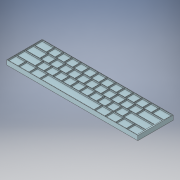
# Autodesk Inventor part: keyboard-base_standard
Saved by Autodesk Inventor 2016 (Build 200138000, 138)
## iProperties
Created: 2016-12-08
Part Number: keyboard-base_standard
Material: Generic
Document SubType Name: Modeling
Designer: Cemra JC
Density: 1 g/cm^3
Appearance: Default
Author: Cemra JC
Autodesk Inventor part; units mm, degrees
ref_plane "YZ Plane" through (0, 0, 0) normal (1, 0, 0) x (0, 1, 0)
ref_plane "XZ Plane" through (0, 0, 0) normal (0, 1, 0) x (-1, 0, 0)
ref_plane "XY Plane" through (0, 0, 0) normal (0, 0, 1) x (1, 0, 0)
sketch "Keyboard Backplane" plane through (0, 0, 0) normal (0, 1, 0) x (-1, 0, 0)
  line L0 (144, 38.9) -> (-144, 38.9)
  line L1 (-144, 38.9) -> (-144, -38.9)
  line L2 (-144, -38.9) -> (144, -38.9)
  line L3 (144, -38.9) -> (144, 38.9)
  line L4 (144, 38.9) -> (-144, -38.9) construction
  line L5 (-144, 38.9) -> (144, -38.9) construction
  point P0 (0, 0)
  point P1 (0, 0)
  dimension "d0" = 77.8
  dimension "d1" = 288
  constraints: 12 end point, 2 parallel, 1 coincident, 1 horizontal, 1 midpoint, 1 perpendicular
  measures "d0" distance of L0.end L1.end
  measures "d1" distance of L1.end L2.end
extrude "Keyboard Backplane Body" add sketch "Keyboard Backplane" along normal blind 10
sketch "KeyCap Outlines" plane through (0, 10, 0) normal (0, 1, 0) x (1, 0, 0)
  line L0 (-143, 37.9) -> (-115.7, 37.9)
  line L1 (-115.7, 37.9) -> (-115.7, 19.7)
  line L2 (-115.7, 19.7) -> (-143, 19.7)
  line L3 (-143, 19.7) -> (-143, 37.9)
  line L4 (-144, -38.9) -> (144, -38.9) projected
  line L5 (144, -38.9) -> (144, 38.9) projected
  line L6 (144, 38.9) -> (-144, 38.9) projected
  line L7 (-144, 38.9) -> (-144, -38.9) projected
  line L8 (-114.7, 19.7) -> (-96.5, 19.7)
  line L9 (-96.5, 19.7) -> (-96.5, 37.9)
  line L10 (-96.5, 37.9) -> (-114.7, 37.9)
  line L11 (-114.7, 37.9) -> (-114.7, 19.7)
  line L12 (-95.5, 19.7) -> (-77.3, 19.7)
  line L13 (-77.3, 19.7) -> (-77.3, 37.9)
  line L14 (-77.3, 37.9) -> (-95.5, 37.9)
  line L15 (-95.5, 37.9) -> (-95.5, 19.7)
  line L16 (-76.3, 19.7) -> (-58.1, 19.7)
  line L17 (-58.1, 19.7) -> (-58.1, 37.9)
  line L18 (-58.1, 37.9) -> (-76.3, 37.9)
  line L19 (-76.3, 37.9) -> (-76.3, 19.7)
  line L20 (-57.1, 19.7) -> (-38.9, 19.7)
  line L21 (-38.9, 19.7) -> (-38.9, 37.9)
  line L22 (-38.9, 37.9) -> (-57.1, 37.9)
  line L23 (-57.1, 37.9) -> (-57.1, 19.7)
  line L24 (-37.9, 19.7) -> (-19.7, 19.7)
  line L25 (-19.7, 19.7) -> (-19.7, 37.9)
  line L26 (-19.7, 37.9) -> (-37.9, 37.9)
  line L27 (-37.9, 37.9) -> (-37.9, 19.7)
  line L28 (-18.7, 19.7) -> (-0.5, 19.7)
  line L29 (-0.5, 19.7) -> (-0.5, 37.9)
  line L30 (-0.5, 37.9) -> (-18.7, 37.9)
  line L31 (-18.7, 37.9) -> (-18.7, 19.7)
  line L32 (0.5, 19.7) -> (18.7, 19.7)
  line L33 (18.7, 19.7) -> (18.7, 37.9)
  line L34 (18.7, 37.9) -> (0.5, 37.9)
  line L35 (0.5, 37.9) -> (0.5, 19.7)
  line L36 (19.7, 19.7) -> (37.9, 19.7)
  line L37 (37.9, 19.7) -> (37.9, 37.9)
  line L38 (37.9, 37.9) -> (19.7, 37.9)
  line L39 (19.7, 37.9) -> (19.7, 19.7)
  line L40 (38.9, 19.7) -> (57.1, 19.7)
  line L41 (57.1, 19.7) -> (57.1, 37.9)
  line L42 (57.1, 37.9) -> (38.9, 37.9)
  line L43 (38.9, 37.9) -> (38.9, 19.7)
  line L44 (58.1, 19.7) -> (76.3, 19.7)
  line L45 (76.3, 19.7) -> (76.3, 37.9)
  line L46 (76.3, 37.9) -> (58.1, 37.9)
  line L47 (58.1, 37.9) -> (58.1, 19.7)
  line L48 (77.3, 19.7) -> (95.5, 19.7)
  line L49 (95.5, 19.7) -> (95.5, 37.9)
  line L50 (95.5, 37.9) -> (77.3, 37.9)
  line L51 (77.3, 37.9) -> (77.3, 19.7)
  line L52 (96.5, 19.7) -> (114.7, 19.7)
  line L53 (114.7, 19.7) -> (114.7, 37.9)
  line L54 (114.7, 37.9) -> (96.5, 37.9)
  line L55 (96.5, 37.9) -> (96.5, 19.7)
  line L56 (115.7, 37.9) -> (143, 37.9)
  line L57 (143, 37.9) -> (143, 19.7)
  line L58 (143, 19.7) -> (115.7, 19.7)
  line L59 (115.7, 19.7) -> (115.7, 37.9)
  line L60 (-143, 18.7) -> (-111.15, 18.7)
  line L61 (-111.15, 18.7) -> (-111.15, 0.5)
  line L62 (-111.15, 0.5) -> (-143, 0.5)
  line L63 (-143, 0.5) -> (-143, 18.7)
  line L64 (-110.15, 0.5) -> (-91.95, 0.5)
  line L65 (-91.95, 0.5) -> (-91.95, 18.7)
  line L66 (-91.95, 18.7) -> (-110.15, 18.7)
  line L67 (-110.15, 18.7) -> (-110.15, 0.5)
  line L68 (-72.75, 0.5) -> (-72.75, 18.7)
  line L69 (-72.75, 18.7) -> (-90.95, 18.7)
  line L70 (-90.95, 18.7) -> (-90.95, 0.5)
  line L71 (-90.95, 0.5) -> (-72.75, 0.5)
  line L72 (-53.55, 0.5) -> (-53.55, 18.7)
  line L73 (-53.55, 18.7) -> (-71.75, 18.7)
  line L74 (-71.75, 18.7) -> (-71.75, 0.5)
  line L75 (-71.75, 0.5) -> (-53.55, 0.5)
  line L76 (-34.35, 0.5) -> (-34.35, 18.7)
  line L77 (-34.35, 18.7) -> (-52.55, 18.7)
  line L78 (-52.55, 18.7) -> (-52.55, 0.5)
  line L79 (-52.55, 0.5) -> (-34.35, 0.5)
  line L80 (-15.15, 0.5) -> (-15.15, 18.7)
  line L81 (-15.15, 18.7) -> (-33.35, 18.7)
  line L82 (-33.35, 18.7) -> (-33.35, 0.5)
  line L83 (-33.35, 0.5) -> (-15.15, 0.5)
  line L84 (4.05, 0.5) -> (4.05, 18.7)
  line L85 (4.05, 18.7) -> (-14.15, 18.7)
  line L86 (-14.15, 18.7) -> (-14.15, 0.5)
  line L87 (-14.15, 0.5) -> (4.05, 0.5)
  line L88 (23.25, 0.5) -> (23.25, 18.7)
  line L89 (23.25, 18.7) -> (5.05, 18.7)
  line L90 (5.05, 18.7) -> (5.05, 0.5)
  line L91 (5.05, 0.5) -> (23.25, 0.5)
  line L92 (42.45, 0.5) -> (42.45, 18.7)
  line L93 (42.45, 18.7) -> (24.25, 18.7)
  line L94 (24.25, 18.7) -> (24.25, 0.5)
  line L95 (24.25, 0.5) -> (42.45, 0.5)
  line L96 (61.65, 0.5) -> (61.65, 18.7)
  line L97 (61.65, 18.7) -> (43.45, 18.7)
  line L98 (43.45, 18.7) -> (43.45, 0.5)
  line L99 (43.45, 0.5) -> (61.65, 0.5)
  line L100 (80.85, 0.5) -> (80.85, 18.7)
  line L101 (80.85, 18.7) -> (62.65, 18.7)
  line L102 (62.65, 18.7) -> (62.65, 0.5)
  line L103 (62.65, 0.5) -> (80.85, 0.5)
  line L104 (100.05, 0.5) -> (100.05, 18.7)
  line L105 (100.05, 18.7) -> (81.85, 18.7)
  line L106 (81.85, 18.7) -> (81.85, 0.5)
  line L107 (81.85, 0.5) -> (100.05, 0.5)
  line L108 (101.05, 18.7) -> (142, 18.7)
  line L109 (142, 18.7) -> (142, 0.5)
  line L110 (142, 0.5) -> (101.05, 0.5)
  line L111 (101.05, 0.5) -> (101.05, 18.7)
  line L112 (-143, -0.5) -> (-102.05, -0.5)
  line L113 (-102.05, -0.5) -> (-102.05, -18.7)
  line L114 (-102.05, -18.7) -> (-143, -18.7)
  line L115 (-143, -18.7) -> (-143, -0.5)
  line L116 (-101.05, -0.5) -> (-82.85, -0.5)
  line L117 (-82.85, -0.5) -> (-82.85, -18.7)
  line L118 (-82.85, -18.7) -> (-101.05, -18.7)
  line L119 (-101.05, -18.7) -> (-101.05, -0.5)
  line L120 (-63.65, -18.7) -> (-81.85, -18.7)
  line L121 (-63.65, -0.5) -> (-63.65, -18.7)
  line L122 (-81.85, -18.7) -> (-81.85, -0.5)
  line L123 (-81.85, -0.5) -> (-63.65, -0.5)
  line L124 (-44.45, -18.7) -> (-62.65, -18.7)
  line L125 (-44.45, -0.5) -> (-44.45, -18.7)
  line L126 (-62.65, -18.7) -> (-62.65, -0.5)
  line L127 (-62.65, -0.5) -> (-44.45, -0.5)
  line L128 (-25.25, -18.7) -> (-43.45, -18.7)
  line L129 (-25.25, -0.5) -> (-25.25, -18.7)
  line L130 (-43.45, -18.7) -> (-43.45, -0.5)
  line L131 (-43.45, -0.5) -> (-25.25, -0.5)
  line L132 (-6.05, -18.7) -> (-24.25, -18.7)
  line L133 (-6.05, -0.5) -> (-6.05, -18.7)
  line L134 (-24.25, -18.7) -> (-24.25, -0.5)
  line L135 (-24.25, -0.5) -> (-6.05, -0.5)
  line L136 (13.15, -18.7) -> (-5.05, -18.7)
  line L137 (13.15, -0.5) -> (13.15, -18.7)
  line L138 (-5.05, -18.7) -> (-5.05, -0.5)
  line L139 (-5.05, -0.5) -> (13.15, -0.5)
  line L140 (32.35, -18.7) -> (14.15, -18.7)
  line L141 (32.35, -0.5) -> (32.35, -18.7)
  line L142 (14.15, -18.7) -> (14.15, -0.5)
  line L143 (14.15, -0.5) -> (32.35, -0.5)
  line L144 (51.55, -18.7) -> (33.35, -18.7)
  line L145 (51.55, -0.5) -> (51.55, -18.7)
  line L146 (33.35, -18.7) -> (33.35, -0.5)
  line L147 (33.35, -0.5) -> (51.55, -0.5)
  line L148 (70.75, -18.7) -> (52.55, -18.7)
  line L149 (70.75, -0.5) -> (70.75, -18.7)
  line L150 (52.55, -18.7) -> (52.55, -0.5)
  line L151 (52.55, -0.5) -> (70.75, -0.5)
  line L152 (89.95, -18.7) -> (71.75, -18.7)
  line L153 (89.95, -0.5) -> (89.95, -18.7)
  line L154 (71.75, -18.7) -> (71.75, -0.5)
  line L155 (71.75, -0.5) -> (89.95, -0.5)
  line L156 (90.95, -18.7) -> (141, -18.7)
  line L157 (141, -18.7) -> (141, -0.5)
  line L158 (141, -0.5) -> (90.95, -0.5)
  line L159 (90.95, -0.5) -> (90.95, -18.7)
  line L160 (-143, -37.9) -> (-120.25, -37.9)
  line L161 (-120.25, -37.9) -> (-120.25, -19.7)
  line L162 (-120.25, -19.7) -> (-143, -19.7)
  line L163 (-143, -19.7) -> (-143, -37.9)
  line L164 (-143, -37.9) -> (-120.25, -19.7) construction
  line L165 (-120.25, -37.9) -> (-143, -19.7) construction
  line L166 (-96.5, -37.9) -> (-96.5, -19.7)
  line L167 (-96.5, -19.7) -> (-119.25, -19.7)
  line L168 (-119.25, -19.7) -> (-119.25, -37.9)
  line L169 (-119.25, -37.9) -> (-96.5, -37.9)
  line L170 (-72.75, -37.9) -> (-72.75, -19.7)
  line L171 (-72.75, -19.7) -> (-95.5, -19.7)
  line L172 (-95.5, -19.7) -> (-95.5, -37.9)
  line L173 (-95.5, -37.9) -> (-72.75, -37.9)
  line L174 (-71.75, -19.7) -> (46.55, -19.7)
  line L175 (46.55, -19.7) -> (46.55, -37.9)
  line L176 (46.55, -37.9) -> (-71.75, -37.9)
  line L177 (-71.75, -37.9) -> (-71.75, -19.7)
  line L178 (47.55, -19.7) -> (70.3, -19.7)
  line L179 (70.3, -19.7) -> (70.3, -37.9)
  line L180 (70.3, -37.9) -> (47.55, -37.9)
  line L181 (47.55, -37.9) -> (47.55, -19.7)
  line L182 (94.05, -37.9) -> (71.3, -37.9)
  line L183 (71.3, -37.9) -> (71.3, -19.7)
  line L184 (71.3, -19.7) -> (94.05, -19.7)
  line L185 (94.05, -19.7) -> (94.05, -37.9)
  line L186 (117.8, -37.9) -> (95.05, -37.9)
  line L187 (95.05, -37.9) -> (95.05, -19.7)
  line L188 (95.05, -19.7) -> (117.8, -19.7)
  line L189 (117.8, -19.7) -> (117.8, -37.9)
  line L190 (141.55, -37.9) -> (118.8, -37.9)
  line L191 (118.8, -37.9) -> (118.8, -19.7)
  line L192 (118.8, -19.7) -> (141.55, -19.7)
  line L193 (141.55, -19.7) -> (141.55, -37.9)
  point P0 (0, 0)
  point P1 (-131.625, -28.8)
  dimension "d4" = 27.3
  dimension "d5" = 18.2
  dimension "d6" = 1
  dimension "d7" = 1
  dimension "d8" = 18.2
  dimension "d9" = 18.2
  dimension "d10" = 1
  dimension "d11" = 1
  dimension "d14" = 19.2
  dimension "d19" = 27.3
  dimension "d20" = 18.2
  dimension "d21" = 1
  dimension "d22" = 1
  dimension "d23" = 18.2
  dimension "d24" = 31.85
  dimension "d25" = 1
  dimension "d26" = 1
  dimension "d27" = 18.2
  dimension "d28" = 18.2
  dimension "d29" = 1
  dimension "d30" = 1
  dimension "d33" = 19.2
  dimension "d38" = 18.2
  dimension "d39" = 40.95
  dimension "d40" = 1
  dimension "d41" = 1
  dimension "d42" = 18.2
  dimension "d43" = 40.95
  dimension "d44" = 1
  dimension "d45" = 1
  dimension "d46" = 18.2
  dimension "d47" = 18.2
  dimension "d48" = 1
  dimension "d49" = 1
  dimension "d52" = 19.2
  dimension "d57" = 18.2
  dimension "d58" = 50.05
  dimension "d59" = 1
  dimension "d60" = 1
  dimension "d63" = 22.75
  dimension "d64" = 18.2
  dimension "d65" = 1
  dimension "d66" = 1
  dimension "d69" = 23.75
  dimension "d74" = 118.3
  dimension "d75" = 18.2
  dimension "d76" = 1
  dimension "d77" = 1
  dimension "d78" = 22.75
  dimension "d79" = 18.2
  dimension "d80" = 1
  dimension "d81" = 1
  dimension "d84" = 23.75
  constraints: 380 end point, 24 parallel, 17 horizontal, 12 perpendicular, 5 collinear, 2 midpoint, 275 other
  measures "d4" distance of L1.end L2.end
  measures "d5" distance of L0.end L1.end
  measures "d6" distance between parallel lines of L6 L0
  measures "d7" distance between parallel lines of L7 L3
  measures "d8" distance of L10.end L9.end
  measures "d9" distance of L9.end L8.end
  measures "d10" distance between parallel lines of L6 L10
  measures "d11" distance between parallel lines of L1 L11
  measures "d14" distance of L8.start L12.start
  measures "d19" distance of L57.end L58.end
  measures "d20" distance of L56.end L57.end
  measures "d21" distance between parallel lines of L6 L56
  measures "d22" distance between parallel lines of L53 L59
  measures "d23" distance of L60.end L61.end
  measures "d24" distance of L61.end L62.end
  measures "d25" distance between parallel lines of L2 L60
  measures "d26" distance between parallel lines of L7 L63
  measures "d27" distance of L65.end L66.end
  measures "d28" distance of L64.end L65.end
  measures "d29" distance between parallel lines of L8 L66
  measures "d30" distance between parallel lines of L61 L67
  measures "d33" distance of L64.end L68.start
  measures "d38" distance of L108.end L109.end
  measures "d39" distance of L109.end L110.end
  measures "d40" distance between parallel lines of L104 L111
  measures "d41" distance between parallel lines of L58 L108
  measures "d42" distance of L112.end L113.end
  measures "d43" distance of L113.end L114.end
  measures "d44" distance between parallel lines of L7 L115
  measures "d45" distance between parallel lines of L62 L112
  measures "d46" distance of L116.end L117.end
  measures "d47" distance of L117.end L118.end
  measures "d48" distance between parallel lines of L113 L119
  measures "d49" distance between parallel lines of L64 L116
  measures "d52" distance of L117.end L120.start
  measures "d57" distance of L156.end L157.end
  measures "d58" distance of L156.start L156.end
  measures "d59" distance between parallel lines of L153 L159
  measures "d60" distance between parallel lines of L110 L158
  measures "d63" distance of L162.end L161.end
  measures "d64" distance of L161.end L160.end
  measures "d65" distance between parallel lines of L114 L162
  measures "d66" distance between parallel lines of L7 L163
  measures "d69" distance of L160.end L166.start
  measures "d74" distance of L175.end L176.end
  measures "d75" distance of L174.end L175.end
  measures "d76" distance between parallel lines of L170 L177
  measures "d77" distance between parallel lines of L120 L174
  measures "d78" distance of L179.end L180.end
  measures "d79" distance of L178.end L179.end
  measures "d80" distance between parallel lines of L144 L178
  measures "d81" distance between parallel lines of L175 L181
  measures "d84" distance of L179.end L182.start
extrude "Keycap Holes" cut sketch "KeyCap Outlines" against normal blind 3 contours L0 L1 L2 L3 | L11 L10 L9 L8 | L15 L14 L13 L12 | L19 L18 L17 L16 | L23 L22 L21 L20 | L27 L26 L25 L24 | L31 L30 L29 L28 | L35 L34 L33 L32 | L39 L38 L37 L36 | L43 L42 L41 L40 | L47 L46 L45 L44 | L51 L50 L49 L48 | L55 L54 L53 L52 | L56 L57 L58 L59 | L60 L61 L62 L63 | L67 L66 L65 L64 | L71 L70 L69 L68 | L75 L74 L73 L72 | L79 L78 L77 L76 | L83 L82 L81 L80 | L87 L86 L85 L84 | L91 L90 L89 L88 | L95 L94 L93 L92 | L99 L98 L97 L96 | L103 L102 L101 L100 | L107 L106 L105 L104 | L108 L109 L110 L111 | L112 L113 L114 L115 | L116 L117 L118 L119 | L120 L122 L123 L121 | L124 L126 L127 L125 | L128 L130 L131 L129 | L132 L134 L135 L133 | L136 L138 L139 L137 | L140 L142 L143 L141 | L144 L146 L147 L145 | L148 L150 L151 L149 | L152 L154 L155 L153 | L159 L158 L157 L156 | L163 L162 L161 L160 | L169 L168 L167 L166 | L173 L172 L171 L170 | L174 L175 L176 L177 | L178 L179 L180 L181 | L182 L183 L184 L185 | L186 L187 L188 L189 | L190 L191 L192 L193
equation "\"d0\" = b_height"
equation "\"d1\" = b_width"
equation "\"d4\" = b_tab"
equation "\"d5\" = k_width"
equation "\"d6\" = d7"
equation "\"d7\" = b_pad"
equation "\"d8\" = d5"
equation "\"d9\" = d5"
equation "\"d10\" = d6"
equation "\"d11\" = d7"
equation "\"d14\" = d8 + b_pad"
equation "\"d19\" = d4"
equation "\"d20\" = d5"
equation "\"d21\" = d7"
equation "\"d22\" = d7"
equation "\"d23\" = d5"
equation "\"d24\" = b_caps"
equation "\"d25\" = d7"
equation "\"d26\" = d7"
equation "\"d27\" = d5"
equation "\"d28\" = d5"
equation "\"d29\" = b_pad"
equation "\"d30\" = d29"
equation "\"d33\" = d27 + d7"
equation "\"d38\" = d5"
equation "\"d39\" = b_lshift"
equation "\"d40\" = d7"
equation "\"d41\" = d7"
equation "\"d42\" = d5"
equation "\"d43\" = d39"
equation "\"d44\" = d7"
equation "\"d45\" = d7"
equation "\"d46\" = d5"
equation "\"d47\" = d5"
equation "\"d48\" = d7"
equation "\"d49\" = d7"
equation "\"d52\" = d47 + d48"
equation "\"d57\" = d5"
equation "\"d58\" = b_rshift"
equation "\"d59\" = d7"
equation "\"d60\" = d7"
equation "\"d63\" = b_ctrl"
equation "\"d64\" = d5"
equation "\"d65\" = d7"
equation "\"d66\" = d7"
equation "\"d69\" = b_ctrl + b_pad"
equation "\"d74\" = b_space"
equation "\"d75\" = d5"
equation "\"d76\" = d7"
equation "\"d77\" = d7"
equation "\"d78\" = b_ctrl"
equation "\"d79\" = k_width"
equation "\"d80\" = d7"
equation "\"d81\" = d7"
equation "\"d84\" = b_ctrl + b_pad"
equation "\"k_width\" = 18.2"
equation "\"k_height\" = 16.5"
equation "\"k_taper1\" = 1.5"
equation "\"k_taper2\" = 0.5"
equation "\"k_radius\" = 6"
equation "\"k_wthick\" = 1.5"
equation "\"k_ribthick\" = 1.5"
equation "\"k_ribheight\" = 5"
equation "\"k_poleoff\" = 2.275"
equation "\"k_poledia\" = 5.3"
equation "\"k_cmxw\" = 1.55"
equation "\"k_cmxl\" = 4.35"
equation "\"s_bwidth\" = 14.4"
equation "\"s_poleh\" = 3.6"
equation "\"s_polebw\" = 5.4"
equation "\"s_polebl\" = 7.45"
equation "\"b_pad\" = 1"
equation "\"b_tab\" = 27.3"
equation "\"b_caps\" = 31.85"
equation "\"b_lshift\" = 40.95"
equation "\"b_rshift\" = 50.05"
equation "\"b_ctrl\" = 22.75"
equation "\"b_space\" = 118.3"
equation "\"b_width\" = 288"
equation "\"b_height\" = 77.8"
equation "\"k_staper\" = 1"
equation "\"k_ltaper\" = 1.5"
equation "\"k_lradius\" = 6"
equation "\"k_sradius\" = 4"
equation "\"k_height_t\" = 16"
equation "\"k_taper_wide\" = 1.5"
equation "\"k_height_low\" = 15"
equation "\"k_taper_thin\" = 0.5"
equation "\"k_shortening\" = 4.5"
equation "\"k_cmxd\" = 4"
body "Solid1"
